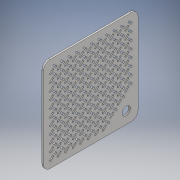
# Autodesk Inventor part: ExtrusionFrontpanel2
Saved by Autodesk Inventor 2017 (Build 210142000, 142)
## iProperties
Created: 2019-06-19
Part Number: ExtrusionFrontpanel2
Material: Generic
Document SubType Name: Modeling
Designer: DDeGo
Density: 1 g/cm^3
Appearance: Default
Author: DDeGo
Autodesk Inventor part; units mm, degrees
(part 1 of 3)
ref_plane "YZ Plane" through (0, 0, 0) normal (1, 0, 0) x (0, 1, 0)
ref_plane "XZ Plane" through (0, 0, 0) normal (0, 1, 0) x (-1, 0, 0)
ref_plane "XY Plane" through (0, 0, 0) normal (0, 0, 1) x (1, 0, 0)
sketch "Sketch1" plane through (0, 0, 0) normal (1, 0, 0) x (0, 1, 0)
  line L0 (0, 13) -> (157, 13)
  line L1 (170, 0) -> (170, -157)
  line L2 (157, -170) -> (0, -170)
  line L3 (-13, -157) -> (-13, 0)
  arc A0 (170, 0) -> (157, 13) centre (157, 0) ccw
  arc A1 (157, -170) -> (170, -157) centre (157, -157) ccw
  arc A2 (-13, -157) -> (0, -170) centre (0, -157) ccw
  arc A3 (0, 13) -> (-13, 0) centre (0, 0) ccw
  point P0 (-13, 13)
  dimension "d0" = 183
  dimension "d1" = 183
  dimension "d4" = 13
  constraints: 8 end point, 8 point on circle, 8 tangent, 4 centre point, 3 equal radius, 2 parallel, 2 point on line, 1 coincident, 1 horizontal, 1 perpendicular
  measures "d0" distance between parallel lines of L2 L0
  measures "d1" distance between parallel lines of L3 L1
  measures "d4" radius of A0
extrude "Extrusion1" add sketch "Sketch1" along normal blind 3
sketch "Sketch7" plane through (3, 0, 0) normal (1, 0, 0) x (0, 0, -1)
  arc A0 (170, 157) -> (157, 170) centre (157, 157) ccw construction
  line L0 (0, 0) -> (157, 0) construction
  line L1 (157, 0) -> (157, 157) construction
  line L2 (157, 157) -> (0, 157) construction
  line L3 (0, 157) -> (0, 0) construction
  line L4 (157, 0) -> (152, 5) construction
  line L5 (158.0607, 1.0607) -> (153.0607, 6.0607)
  line L6 (150.9393, 3.9393) -> (155.9393, -1.0607)
  arc A1 (155.9393, -1.0607) -> (158.0607, 1.0607) centre (157, 0) ccw
  arc A2 (153.0607, 6.0607) -> (150.9393, 3.9393) centre (152, 5) ccw
  line L7 (150.3787, 11.6213) -> (145.3787, 6.6213) construction
  line L8 (151.4393, 10.5607) -> (146.4393, 5.5607)
  line L9 (144.318, 7.682) -> (149.318, 12.682)
  arc A3 (151.4393, 10.5607) -> (149.318, 12.682) centre (150.3787, 11.6213) ccw
  arc A4 (144.318, 7.682) -> (146.4393, 5.5607) centre (145.3787, 6.6213) ccw
  line L10 (148.9393, 8.0607) -> (150.9393, 6.0607) construction
  line L11 (157, 14.5379) -> (152, 19.5379) construction
  line L12 (150.9393, 18.4772) -> (155.9393, 13.4772)
  arc A5 (155.9393, 13.4772) -> (158.0607, 15.5985) centre (157, 14.5379) ccw
  line L13 (158.0607, 15.5985) -> (153.0607, 20.5985)
  arc A6 (153.0607, 20.5985) -> (150.9393, 18.4772) centre (152, 19.5379) ccw
  line L14 (148.9393, 22.5985) -> (150.9393, 20.5985) construction
  line L15 (151.4393, 25.0985) -> (146.4393, 20.0985)
  arc A7 (144.318, 22.2198) -> (146.4393, 20.0985) centre (145.3787, 21.1592) ccw
  line L16 (150.3787, 26.1592) -> (145.3787, 21.1592) construction
  line L17 (144.318, 22.2198) -> (149.318, 27.2198)
  arc A8 (151.4393, 25.0985) -> (149.318, 27.2198) centre (150.3787, 26.1592) ccw
  line L18 (157, 29.0757) -> (152, 34.0757) construction
  line L19 (150.9393, 33.0151) -> (155.9393, 28.0151)
  arc A9 (155.9393, 28.0151) -> (158.0607, 30.1364) centre (157, 29.0757) ccw
  line L20 (158.0607, 30.1364) -> (153.0607, 35.1364)
  arc A10 (153.0607, 35.1364) -> (150.9393, 33.0151) centre (152, 34.0757) ccw
  line L21 (148.9393, 37.1364) -> (150.9393, 35.1364) construction
  line L22 (151.4393, 39.6364) -> (146.4393, 34.6364)
  arc A11 (144.318, 36.7577) -> (146.4393, 34.6364) centre (145.3787, 35.6971) ccw
  line L23 (150.3787, 40.6971) -> (145.3787, 35.6971) construction
  line L24 (144.318, 36.7577) -> (149.318, 41.7577)
  arc A12 (151.4393, 39.6364) -> (149.318, 41.7577) centre (150.3787, 40.6971) ccw
  line L25 (157, 43.6136) -> (152, 48.6136) construction
  line L26 (150.9393, 47.5529) -> (155.9393, 42.5529)
  arc A13 (155.9393, 42.5529) -> (158.0607, 44.6743) centre (157, 43.6136) ccw
  line L27 (158.0607, 44.6743) -> (153.0607, 49.6743)
  arc A14 (153.0607, 49.6743) -> (150.9393, 47.5529) centre (152, 48.6136) ccw
  line L28 (148.9393, 51.6743) -> (150.9393, 49.6743) construction
  line L29 (151.4393, 54.1743) -> (146.4393, 49.1743)
  arc A15 (144.318, 51.2956) -> (146.4393, 49.1743) centre (145.3787, 50.2349) ccw
  line L30 (150.3787, 55.2349) -> (145.3787, 50.2349) construction
  line L31 (144.318, 51.2956) -> (149.318, 56.2956)
  arc A16 (151.4393, 54.1743) -> (149.318, 56.2956) centre (150.3787, 55.2349) ccw
  line L32 (157, 58.1515) -> (152, 63.1515) construction
  line L33 (150.9393, 62.0908) -> (155.9393, 57.0908)
  arc A17 (155.9393, 57.0908) -> (158.0607, 59.2121) centre (157, 58.1515) ccw
  line L34 (158.0607, 59.2121) -> (153.0607, 64.2121)
  arc A18 (153.0607, 64.2121) -> (150.9393, 62.0908) centre (152, 63.1515) ccw
  line L35 (148.9393, 66.2121) -> (150.9393, 64.2121) construction
  line L36 (151.4393, 68.7121) -> (146.4393, 63.7121)
  arc A19 (144.318, 65.8335) -> (146.4393, 63.7121) centre (145.3787, 64.7728) ccw
  line L37 (150.3787, 69.7728) -> (145.3787, 64.7728) construction
  line L38 (144.318, 65.8335) -> (149.318, 70.8335)
  arc A20 (151.4393, 68.7121) -> (149.318, 70.8335) centre (150.3787, 69.7728) ccw
  line L39 (157, 72.6893) -> (152, 77.6893) construction
  line L40 (150.9393, 76.6287) -> (155.9393, 71.6287)
  arc A21 (155.9393, 71.6287) -> (158.0607, 73.75) centre (157, 72.6893) ccw
  line L41 (158.0607, 73.75) -> (153.0607, 78.75)
  arc A22 (153.0607, 78.75) -> (150.9393, 76.6287) centre (152, 77.6893) ccw
  line L42 (148.9393, 80.75) -> (150.9393, 78.75) construction
  line L43 (151.4393, 83.25) -> (146.4393, 78.25)
  arc A23 (144.318, 80.3713) -> (146.4393, 78.25) centre (145.3787, 79.3107) ccw
  line L44 (150.3787, 84.3107) -> (145.3787, 79.3107) construction
  line L45 (144.318, 80.3713) -> (149.318, 85.3713)
  arc A24 (151.4393, 83.25) -> (149.318, 85.3713) centre (150.3787, 84.3107) ccw
  line L46 (157, 87.2272) -> (152, 92.2272) construction
  line L47 (150.9393, 91.1665) -> (155.9393, 86.1665)
  arc A25 (155.9393, 86.1665) -> (158.0607, 88.2879) centre (157, 87.2272) ccw
  line L48 (158.0607, 88.2879) -> (153.0607, 93.2879)
  arc A26 (153.0607, 93.2879) -> (150.9393, 91.1665) centre (152, 92.2272) ccw
  line L49 (148.9393, 95.2879) -> (150.9393, 93.2879) construction
  line L50 (151.4393, 97.7879) -> (146.4393, 92.7879)
  arc A27 (144.318, 94.9092) -> (146.4393, 92.7879) centre (145.3787, 93.8485) ccw
  line L51 (150.3787, 98.8485) -> (145.3787, 93.8485) construction
  line L52 (144.318, 94.9092) -> (149.318, 99.9092)
  arc A28 (151.4393, 97.7879) -> (149.318, 99.9092) centre (150.3787, 98.8485) ccw
  line L53 (157, 101.7651) -> (152, 106.7651) construction
  line L54 (150.9393, 105.7044) -> (155.9393, 100.7044)
  arc A29 (155.9393, 100.7044) -> (158.0607, 102.8257) centre (157, 101.7651) ccw
  line L55 (158.0607, 102.8257) -> (153.0607, 107.8257)
  arc A30 (153.0607, 107.8257) -> (150.9393, 105.7044) centre (152, 106.7651) ccw
  line L56 (148.9393, 109.8257) -> (150.9393, 107.8257) construction
  line L57 (151.4393, 112.3257) -> (146.4393, 107.3257)
  arc A31 (144.318, 109.4471) -> (146.4393, 107.3257) centre (145.3787, 108.3864) ccw
  line L58 (150.3787, 113.3864) -> (145.3787, 108.3864) construction
  line L59 (144.318, 109.4471) -> (149.318, 114.4471)
  arc A32 (151.4393, 112.3257) -> (149.318, 114.4471) centre (150.3787, 113.3864) ccw
  line L60 (157, 116.3029) -> (152, 121.3029) construction
  line L61 (150.9393, 120.2423) -> (155.9393, 115.2423)
  arc A33 (155.9393, 115.2423) -> (158.0607, 117.3636) centre (157, 116.3029) ccw
  line L62 (158.0607, 117.3636) -> (153.0607, 122.3636)
  arc A34 (153.0607, 122.3636) -> (150.9393, 120.2423) centre (152, 121.3029) ccw
  line L63 (148.9393, 124.3636) -> (150.9393, 122.3636) construction
  line L64 (151.4393, 126.8636) -> (146.4393, 121.8636)
  arc A35 (144.318, 123.9849) -> (146.4393, 121.8636) centre (145.3787, 122.9243) ccw
  line L65 (150.3787, 127.9243) -> (145.3787, 122.9243) construction
  line L66 (144.318, 123.9849) -> (149.318, 128.9849)
  arc A36 (151.4393, 126.8636) -> (149.318, 128.9849) centre (150.3787, 127.9243) ccw
  line L67 (157, 130.8408) -> (152, 135.8408) construction
  line L68 (150.9393, 134.7802) -> (155.9393, 129.7802)
  arc A37 (155.9393, 129.7802) -> (158.0607, 131.9015) centre (157, 130.8408) ccw
  line L69 (158.0607, 131.9015) -> (153.0607, 136.9015)
  arc A38 (153.0607, 136.9015) -> (150.9393, 134.7802) centre (152, 135.8408) ccw
  line L70 (148.9393, 138.9015) -> (150.9393, 136.9015) construction
  line L71 (151.4393, 141.4015) -> (146.4393, 136.4015)
  arc A39 (144.318, 138.5228) -> (146.4393, 136.4015) centre (145.3787, 137.4621) ccw
  line L72 (150.3787, 142.4621) -> (145.3787, 137.4621) construction
  line L73 (144.318, 138.5228) -> (149.318, 143.5228)
  arc A40 (151.4393, 141.4015) -> (149.318, 143.5228) centre (150.3787, 142.4621) ccw
  line L74 (157, 145.3787) -> (152, 150.3787) construction
  line L75 (150.9393, 149.318) -> (155.9393, 144.318)
  arc A41 (155.9393, 144.318) -> (158.0607, 146.4393) centre (157, 145.3787) ccw
  line L76 (158.0607, 146.4393) -> (153.0607, 151.4393)
  arc A42 (153.0607, 151.4393) -> (150.9393, 149.318) centre (152, 150.3787) ccw
  line L77 (148.9393, 153.4393) -> (150.9393, 151.4393) construction
  line L78 (151.4393, 155.9393) -> (146.4393, 150.9393)
  arc A43 (144.318, 153.0607) -> (146.4393, 150.9393) centre (145.3787, 152) ccw
  line L79 (150.3787, 157) -> (145.3787, 152) construction
  line L80 (144.318, 153.0607) -> (149.318, 158.0607)
  arc A44 (151.4393, 155.9393) -> (149.318, 158.0607) centre (150.3787, 157) ccw
  line L81 (142.4621, 0) -> (137.4621, 5) construction
  line L82 (136.4015, 3.9393) -> (141.4015, -1.0607)
  arc A45 (141.4015, -1.0607) -> (143.5228, 1.0607) centre (142.4621, 0) ccw
  line L83 (143.5228, 1.0607) -> (138.5228, 6.0607)
  arc A46 (138.5228, 6.0607) -> (136.4015, 3.9393) centre (137.4621, 5) ccw
  line L84 (134.4015, 8.0607) -> (136.4015, 6.0607) construction
  line L85 (136.9015, 10.5607) -> (131.9015, 5.5607)
  arc A47 (129.7802, 7.682) -> (131.9015, 5.5607) centre (130.8408, 6.6213) ccw
  line L86 (135.8408, 11.6213) -> (130.8408, 6.6213) construction
  line L87 (129.7802, 7.682) -> (134.7802, 12.682)
  arc A48 (136.9015, 10.5607) -> (134.7802, 12.682) centre (135.8408, 11.6213) ccw
  line L88 (142.4621, 14.5379) -> (137.4621, 19.5379) construction
  line L89 (136.4015, 18.4772) -> (141.4015, 13.4772)
  arc A49 (141.4015, 13.4772) -> (143.5228, 15.5985) centre (142.4621, 14.5379) ccw
  line L90 (143.5228, 15.5985) -> (138.5228, 20.5985)
  arc A50 (138.5228, 20.5985) -> (136.4015, 18.4772) centre (137.4621, 19.5379) ccw
  line L91 (134.4015, 22.5985) -> (136.4015, 20.5985) construction
  line L92 (136.9015, 25.0985) -> (131.9015, 20.0985)
  arc A51 (129.7802, 22.2198) -> (131.9015, 20.0985) centre (130.8408, 21.1592) ccw
  line L93 (135.8408, 26.1592) -> (130.8408, 21.1592) construction
  line L94 (129.7802, 22.2198) -> (134.7802, 27.2198)
  arc A52 (136.9015, 25.0985) -> (134.7802, 27.2198) centre (135.8408, 26.1592) ccw
  line L95 (142.4621, 29.0757) -> (137.4621, 34.0757) construction
  line L96 (136.4015, 33.0151) -> (141.4015, 28.0151)
  arc A53 (141.4015, 28.0151) -> (143.5228, 30.1364) centre (142.4621, 29.0757) ccw
  line L97 (143.5228, 30.1364) -> (138.5228, 35.1364)
  arc A54 (138.5228, 35.1364) -> (136.4015, 33.0151) centre (137.4621, 34.0757) ccw
  line L98 (134.4015, 37.1364) -> (136.4015, 35.1364) construction
  line L99 (136.9015, 39.6364) -> (131.9015, 34.6364)
  arc A55 (129.7802, 36.7577) -> (131.9015, 34.6364) centre (130.8408, 35.6971) ccw
  line L100 (135.8408, 40.6971) -> (130.8408, 35.6971) construction
  line L101 (129.7802, 36.7577) -> (134.7802, 41.7577)
  arc A56 (136.9015, 39.6364) -> (134.7802, 41.7577) centre (135.8408, 40.6971) ccw
  line L102 (142.4621, 43.6136) -> (137.4621, 48.6136) construction
  line L103 (136.4015, 47.5529) -> (141.4015, 42.5529)
  arc A57 (141.4015, 42.5529) -> (143.5228, 44.6743) centre (142.4621, 43.6136) ccw
  line L104 (143.5228, 44.6743) -> (138.5228, 49.6743)
  arc A58 (138.5228, 49.6743) -> (136.4015, 47.5529) centre (137.4621, 48.6136) ccw
  line L105 (134.4015, 51.6743) -> (136.4015, 49.6743) construction
  line L106 (136.9015, 54.1743) -> (131.9015, 49.1743)
  arc A59 (129.7802, 51.2956) -> (131.9015, 49.1743) centre (130.8408, 50.2349) ccw
  line L107 (135.8408, 55.2349) -> (130.8408, 50.2349) construction
  line L108 (129.7802, 51.2956) -> (134.7802, 56.2956)
  arc A60 (136.9015, 54.1743) -> (134.7802, 56.2956) centre (135.8408, 55.2349) ccw
  line L109 (142.4621, 58.1515) -> (137.4621, 63.1515) construction
  line L110 (136.4015, 62.0908) -> (141.4015, 57.0908)
  arc A61 (141.4015, 57.0908) -> (143.5228, 59.2121) centre (142.4621, 58.1515) ccw
  line L111 (143.5228, 59.2121) -> (138.5228, 64.2121)
  arc A62 (138.5228, 64.2121) -> (136.4015, 62.0908) centre (137.4621, 63.1515) ccw
  line L112 (134.4015, 66.2121) -> (136.4015, 64.2121) construction
  line L113 (136.9015, 68.7121) -> (131.9015, 63.7121)
  arc A63 (129.7802, 65.8335) -> (131.9015, 63.7121) centre (130.8408, 64.7728) ccw
  line L114 (135.8408, 69.7728) -> (130.8408, 64.7728) construction
  line L115 (129.7802, 65.8335) -> (134.7802, 70.8335)
  arc A64 (136.9015, 68.7121) -> (134.7802, 70.8335) centre (135.8408, 69.7728) ccw
  line L116 (142.4621, 72.6893) -> (137.4621, 77.6893) construction
  line L117 (136.4015, 76.6287) -> (141.4015, 71.6287)
  arc A65 (141.4015, 71.6287) -> (143.5228, 73.75) centre (142.4621, 72.6893) ccw
  line L118 (143.5228, 73.75) -> (138.5228, 78.75)
  arc A66 (138.5228, 78.75) -> (136.4015, 76.6287) centre (137.4621, 77.6893) ccw
  line L119 (134.4015, 80.75) -> (136.4015, 78.75) construction
  line L120 (136.9015, 83.25) -> (131.9015, 78.25)
  arc A67 (129.7802, 80.3713) -> (131.9015, 78.25) centre (130.8408, 79.3107) ccw
  line L121 (135.8408, 84.3107) -> (130.8408, 79.3107) construction
  line L122 (129.7802, 80.3713) -> (134.7802, 85.3713)
  arc A68 (136.9015, 83.25) -> (134.7802, 85.3713) centre (135.8408, 84.3107) ccw
  line L123 (142.4621, 87.2272) -> (137.4621, 92.2272) construction
  line L124 (136.4015, 91.1665) -> (141.4015, 86.1665)
  arc A69 (141.4015, 86.1665) -> (143.5228, 88.2879) centre (142.4621, 87.2272) ccw
  line L125 (143.5228, 88.2879) -> (138.5228, 93.2879)
  arc A70 (138.5228, 93.2879) -> (136.4015, 91.1665) centre (137.4621, 92.2272) ccw
  line L126 (134.4015, 95.2879) -> (136.4015, 93.2879) construction
  line L127 (136.9015, 97.7879) -> (131.9015, 92.7879)
  arc A71 (129.7802, 94.9092) -> (131.9015, 92.7879) centre (130.8408, 93.8485) ccw
  line L128 (135.8408, 98.8485) -> (130.8408, 93.8485) construction
  line L129 (129.7802, 94.9092) -> (134.7802, 99.9092)
  arc A72 (136.9015, 97.7879) -> (134.7802, 99.9092) centre (135.8408, 98.8485) ccw
  line L130 (142.4621, 101.7651) -> (137.4621, 106.7651) construction
  line L131 (136.4015, 105.7044) -> (141.4015, 100.7044)
  arc A73 (141.4015, 100.7044) -> (143.5228, 102.8257) centre (142.4621, 101.7651) ccw
  line L132 (143.5228, 102.8257) -> (138.5228, 107.8257)
  arc A74 (138.5228, 107.8257) -> (136.4015, 105.7044) centre (137.4621, 106.7651) ccw
  line L133 (134.4015, 109.8257) -> (136.4015, 107.8257) construction
  line L134 (136.9015, 112.3257) -> (131.9015, 107.3257)
  arc A75 (129.7802, 109.4471) -> (131.9015, 107.3257) centre (130.8408, 108.3864) ccw
  line L135 (135.8408, 113.3864) -> (130.8408, 108.3864) construction
  line L136 (129.7802, 109.4471) -> (134.7802, 114.4471)
  arc A76 (136.9015, 112.3257) -> (134.7802, 114.4471) centre (135.8408, 113.3864) ccw
  line L137 (142.4621, 116.3029) -> (137.4621, 121.3029) construction
  line L138 (136.4015, 120.2423) -> (141.4015, 115.2423)
  arc A77 (141.4015, 115.2423) -> (143.5228, 117.3636) centre (142.4621, 116.3029) ccw
  line L139 (143.5228, 117.3636) -> (138.5228, 122.3636)
  arc A78 (138.5228, 122.3636) -> (136.4015, 120.2423) centre (137.4621, 121.3029) ccw
  line L140 (134.4015, 124.3636) -> (136.4015, 122.3636) construction
  line L141 (136.9015, 126.8636) -> (131.9015, 121.8636)
  arc A79 (129.7802, 123.9849) -> (131.9015, 121.8636) centre (130.8408, 122.9243) ccw
  line L142 (135.8408, 127.9243) -> (130.8408, 122.9243) construction
  line L143 (129.7802, 123.9849) -> (134.7802, 128.9849)
  arc A80 (136.9015, 126.8636) -> (134.7802, 128.9849) centre (135.8408, 127.9243) ccw
  line L144 (142.4621, 130.8408) -> (137.4621, 135.8408) construction
  line L145 (136.4015, 134.7802) -> (141.4015, 129.7802)
  arc A81 (141.4015, 129.7802) -> (143.5228, 131.9015) centre (142.4621, 130.8408) ccw
  line L146 (143.5228, 131.9015) -> (138.5228, 136.9015)
  arc A82 (138.5228, 136.9015) -> (136.4015, 134.7802) centre (137.4621, 135.8408) ccw
  line L147 (134.4015, 138.9015) -> (136.4015, 136.9015) construction
  line L148 (136.9015, 141.4015) -> (131.9015, 136.4015)
  arc A83 (129.7802, 138.5228) -> (131.9015, 136.4015) centre (130.8408, 137.4621) ccw
  line L149 (135.8408, 142.4621) -> (130.8408, 137.4621) construction
  line L150 (129.7802, 138.5228) -> (134.7802, 143.5228)
  arc A84 (136.9015, 141.4015) -> (134.7802, 143.5228) centre (135.8408, 142.4621) ccw
  line L151 (142.4621, 145.3787) -> (137.4621, 150.3787) construction
  line L152 (136.4015, 149.318) -> (141.4015, 144.318)
  arc A85 (141.4015, 144.318) -> (143.5228, 146.4393) centre (142.4621, 145.3787) ccw
  line L153 (143.5228, 146.4393) -> (138.5228, 151.4393)
  arc A86 (138.5228, 151.4393) -> (136.4015, 149.318) centre (137.4621, 150.3787) ccw
  line L154 (134.4015, 153.4393) -> (136.4015, 151.4393) construction
  line L155 (136.9015, 155.9393) -> (131.9015, 150.9393)
  arc A87 (129.7802, 153.0607) -> (131.9015, 150.9393) centre (130.8408, 152) ccw
  line L156 (135.8408, 157) -> (130.8408, 152) construction
  line L157 (129.7802, 153.0607) -> (134.7802, 158.0607)
  arc A88 (136.9015, 155.9393) -> (134.7802, 158.0607) centre (135.8408, 157) ccw
  line L158 (127.9243, 0) -> (122.9243, 5) construction
  line L159 (121.8636, 3.9393) -> (126.8636, -1.0607)
  arc A89 (126.8636, -1.0607) -> (128.9849, 1.0607) centre (127.9243, 0) ccw
  line L160 (128.9849, 1.0607) -> (123.9849, 6.0607)
  arc A90 (123.9849, 6.0607) -> (121.8636, 3.9393) centre (122.9243, 5) ccw
  line L161 (119.8636, 8.0607) -> (121.8636, 6.0607) construction
  line L162 (122.3636, 10.5607) -> (117.3636, 5.5607)
  arc A91 (115.2423, 7.682) -> (117.3636, 5.5607) centre (116.3029, 6.6213) ccw
  line L163 (121.3029, 11.6213) -> (116.3029, 6.6213) construction
  line L164 (115.2423, 7.682) -> (120.2423, 12.682)
  arc A92 (122.3636, 10.5607) -> (120.2423, 12.682) centre (121.3029, 11.6213) ccw
  line L165 (127.9243, 14.5379) -> (122.9243, 19.5379) construction
  line L166 (121.8636, 18.4772) -> (126.8636, 13.4772)
  arc A93 (126.8636, 13.4772) -> (128.9849, 15.5985) centre (127.9243, 14.5379) ccw
  line L167 (128.9849, 15.5985) -> (123.9849, 20.5985)
  arc A94 (123.9849, 20.5985) -> (121.8636, 18.4772) centre (122.9243, 19.5379) ccw
  line L168 (119.8636, 22.5985) -> (121.8636, 20.5985) construction
  line L169 (122.3636, 25.0985) -> (117.3636, 20.0985)
  arc A95 (115.2423, 22.2198) -> (117.3636, 20.0985) centre (116.3029, 21.1592) ccw
  line L170 (121.3029, 26.1592) -> (116.3029, 21.1592) construction
  line L171 (115.2423, 22.2198) -> (120.2423, 27.2198)
  arc A96 (122.3636, 25.0985) -> (120.2423, 27.2198) centre (121.3029, 26.1592) ccw
  line L172 (127.9243, 29.0757) -> (122.9243, 34.0757) construction
  line L173 (121.8636, 33.0151) -> (126.8636, 28.0151)
  arc A97 (126.8636, 28.0151) -> (128.9849, 30.1364) centre (127.9243, 29.0757) ccw
  line L174 (128.9849, 30.1364) -> (123.9849, 35.1364)
  arc A98 (123.9849, 35.1364) -> (121.8636, 33.0151) centre (122.9243, 34.0757) ccw
  line L175 (119.8636, 37.1364) -> (121.8636, 35.1364) construction
  line L176 (122.3636, 39.6364) -> (117.3636, 34.6364)
  arc A99 (115.2423, 36.7577) -> (117.3636, 34.6364) centre (116.3029, 35.6971) ccw
  line L177 (121.3029, 40.6971) -> (116.3029, 35.6971) construction
  line L178 (115.2423, 36.7577) -> (120.2423, 41.7577)
  arc A100 (122.3636, 39.6364) -> (120.2423, 41.7577) centre (121.3029, 40.6971) ccw
  line L179 (127.9243, 43.6136) -> (122.9243, 48.6136) construction
  line L180 (121.8636, 47.5529) -> (126.8636, 42.5529)
  arc A101 (126.8636, 42.5529) -> (128.9849, 44.6743) centre (127.9243, 43.6136) ccw
  line L181 (128.9849, 44.6743) -> (123.9849, 49.6743)
  arc A102 (123.9849, 49.6743) -> (121.8636, 47.5529) centre (122.9243, 48.6136) ccw
  line L182 (119.8636, 51.6743) -> (121.8636, 49.6743) construction
  line L183 (122.3636, 54.1743) -> (117.3636, 49.1743)
  arc A103 (115.2423, 51.2956) -> (117.3636, 49.1743) centre (116.3029, 50.2349) ccw
  line L184 (121.3029, 55.2349) -> (116.3029, 50.2349) construction
  line L185 (115.2423, 51.2956) -> (120.2423, 56.2956)
  arc A104 (122.3636, 54.1743) -> (120.2423, 56.2956) centre (121.3029, 55.2349) ccw
  line L186 (127.9243, 58.1515) -> (122.9243, 63.1515) construction
  line L187 (121.8636, 62.0908) -> (126.8636, 57.0908)
  arc A105 (126.8636, 57.0908) -> (128.9849, 59.2121) centre (127.9243, 58.1515) ccw
  line L188 (128.9849, 59.2121) -> (123.9849, 64.2121)
  arc A106 (123.9849, 64.2121) -> (121.8636, 62.0908) centre (122.9243, 63.1515) ccw
  line L189 (119.8636, 66.2121) -> (121.8636, 64.2121) construction
  line L190 (122.3636, 68.7121) -> (117.3636, 63.7121)
  arc A107 (115.2423, 65.8335) -> (117.3636, 63.7121) centre (116.3029, 64.7728) ccw
  line L191 (121.3029, 69.7728) -> (116.3029, 64.7728) construction
  line L192 (115.2423, 65.8335) -> (120.2423, 70.8335)
  arc A108 (122.3636, 68.7121) -> (120.2423, 70.8335) centre (121.3029, 69.7728) ccw
  line L193 (127.9243, 72.6893) -> (122.9243, 77.6893) construction
  line L194 (121.8636, 76.6287) -> (126.8636, 71.6287)
  arc A109 (126.8636, 71.6287) -> (128.9849, 73.75) centre (127.9243, 72.6893) ccw
  line L195 (128.9849, 73.75) -> (123.9849, 78.75)
  arc A110 (123.9849, 78.75) -> (121.8636, 76.6287) centre (122.9243, 77.6893) ccw
  line L196 (119.8636, 80.75) -> (121.8636, 78.75) construction
  line L197 (122.3636, 83.25) -> (117.3636, 78.25)
  arc A111 (115.2423, 80.3713) -> (117.3636, 78.25) centre (116.3029, 79.3107) ccw
  line L198 (121.3029, 84.3107) -> (116.3029, 79.3107) construction
  line L199 (115.2423, 80.3713) -> (120.2423, 85.3713)
  arc A112 (122.3636, 83.25) -> (120.2423, 85.3713) centre (121.3029, 84.3107) ccw
  line L200 (127.9243, 87.2272) -> (122.9243, 92.2272) construction
  line L201 (121.8636, 91.1665) -> (126.8636, 86.1665)
  arc A113 (126.8636, 86.1665) -> (128.9849, 88.2879) centre (127.9243, 87.2272) ccw
  line L202 (128.9849, 88.2879) -> (123.9849, 93.2879)
  arc A114 (123.9849, 93.2879) -> (121.8636, 91.1665) centre (122.9243, 92.2272) ccw
  line L203 (119.8636, 95.2879) -> (121.8636, 93.2879) construction
  line L204 (122.3636, 97.7879) -> (117.3636, 92.7879)
  arc A115 (115.2423, 94.9092) -> (117.3636, 92.7879) centre (116.3029, 93.8485) ccw
  line L205 (121.3029, 98.8485) -> (116.3029, 93.8485) construction
  line L206 (115.2423, 94.9092) -> (120.2423, 99.9092)
  arc A116 (122.3636, 97.7879) -> (120.2423, 99.9092) centre (121.3029, 98.8485) ccw
  line L207 (127.9243, 101.7651) -> (122.9243, 106.7651) construction
  line L208 (121.8636, 105.7044) -> (126.8636, 100.7044)
  arc A117 (126.8636, 100.7044) -> (128.9849, 102.8257) centre (127.9243, 101.7651) ccw
  line L209 (128.9849, 102.8257) -> (123.9849, 107.8257)
  arc A118 (123.9849, 107.8257) -> (121.8636, 105.7044) centre (122.9243, 106.7651) ccw
  line L210 (119.8636, 109.8257) -> (121.8636, 107.8257) construction
  line L211 (122.3636, 112.3257) -> (117.3636, 107.3257)
  arc A119 (115.2423, 109.4471) -> (117.3636, 107.3257) centre (116.3029, 108.3864) ccw
  line L212 (121.3029, 113.3864) -> (116.3029, 108.3864) construction
  line L213 (115.2423, 109.4471) -> (120.2423, 114.4471)
  arc A120 (122.3636, 112.3257) -> (120.2423, 114.4471) centre (121.3029, 113.3864) ccw
  line L214 (127.9243, 116.3029) -> (122.9243, 121.3029) construction
  line L215 (121.8636, 120.2423) -> (126.8636, 115.2423)
  arc A121 (126.8636, 115.2423) -> (128.9849, 117.3636) centre (127.9243, 116.3029) ccw
  line L216 (128.9849, 117.3636) -> (123.9849, 122.3636)
  arc A122 (123.9849, 122.3636) -> (121.8636, 120.2423) centre (122.9243, 121.3029) ccw
  line L217 (119.8636, 124.3636) -> (121.8636, 122.3636) construction
  line L218 (122.3636, 126.8636) -> (117.3636, 121.8636)
  arc A123 (115.2423, 123.9849) -> (117.3636, 121.8636) centre (116.3029, 122.9243) ccw
  line L219 (121.3029, 127.9243) -> (116.3029, 122.9243) construction
  line L220 (115.2423, 123.9849) -> (120.2423, 128.9849)
  arc A124 (122.3636, 126.8636) -> (120.2423, 128.9849) centre (121.3029, 127.9243) ccw
  line L221 (127.9243, 130.8408) -> (122.9243, 135.8408) construction
  line L222 (121.8636, 134.7802) -> (126.8636, 129.7802)
  arc A125 (126.8636, 129.7802) -> (128.9849, 131.9015) centre (127.9243, 130.8408) ccw
  line L223 (128.9849, 131.9015) -> (123.9849, 136.9015)
  arc A126 (123.9849, 136.9015) -> (121.8636, 134.7802) centre (122.9243, 135.8408) ccw
  line L224 (119.8636, 138.9015) -> (121.8636, 136.9015) construction
  line L225 (122.3636, 141.4015) -> (117.3636, 136.4015)
  arc A127 (115.2423, 138.5228) -> (117.3636, 136.4015) centre (116.3029, 137.4621) ccw
  line L226 (121.3029, 142.4621) -> (116.3029, 137.4621) construction
  line L227 (115.2423, 138.5228) -> (120.2423, 143.5228)
  arc A128 (122.3636, 141.4015) -> (120.2423, 143.5228) centre (121.3029, 142.4621) ccw
  line L228 (127.9243, 145.3787) -> (122.9243, 150.3787) construction
  line L229 (121.8636, 149.318) -> (126.8636, 144.318)
  arc A129 (126.8636, 144.318) -> (128.9849, 146.4393) centre (127.9243, 145.3787) ccw
  line L230 (128.9849, 146.4393) -> (123.9849, 151.4393)
  arc A130 (123.9849, 151.4393) -> (121.8636, 149.318) centre (122.9243, 150.3787) ccw
  line L231 (119.8636, 153.4393) -> (121.8636, 151.4393) construction
  line L232 (122.3636, 155.9393) -> (117.3636, 150.9393)
  arc A131 (115.2423, 153.0607) -> (117.3636, 150.9393) centre (116.3029, 152) ccw
  line L233 (121.3029, 157) -> (116.3029, 152) construction
  line L234 (115.2423, 153.0607) -> (120.2423, 158.0607)
  arc A132 (122.3636, 155.9393) -> (120.2423, 158.0607) centre (121.3029, 157) ccw
  line L235 (113.3864, 0) -> (108.3864, 5) construction
  line L236 (107.3257, 3.9393) -> (112.3257, -1.0607)
  arc A133 (112.3257, -1.0607) -> (114.4471, 1.0607) centre (113.3864, 0) ccw
  line L237 (114.4471, 1.0607) -> (109.4471, 6.0607)
  arc A134 (109.4471, 6.0607) -> (107.3257, 3.9393) centre (108.3864, 5) ccw
  line L238 (105.3257, 8.0607) -> (107.3257, 6.0607) construction
  line L239 (107.8257, 10.5607) -> (102.8257, 5.5607)
  arc A135 (100.7044, 7.682) -> (102.8257, 5.5607) centre (101.7651, 6.6213) ccw
  line L240 (106.7651, 11.6213) -> (101.7651, 6.6213) construction
  line L241 (100.7044, 7.682) -> (105.7044, 12.682)
  arc A136 (107.8257, 10.5607) -> (105.7044, 12.682) centre (106.7651, 11.6213) ccw
  line L242 (113.3864, 14.5379) -> (108.3864, 19.5379) construction
  line L243 (107.3257, 18.4772) -> (112.3257, 13.4772)
  arc A137 (112.3257, 13.4772) -> (114.4471, 15.5985) centre (113.3864, 14.5379) ccw
  line L244 (114.4471, 15.5985) -> (109.4471, 20.5985)
  arc A138 (109.4471, 20.5985) -> (107.3257, 18.4772) centre (108.3864, 19.5379) ccw
  line L245 (105.3257, 22.5985) -> (107.3257, 20.5985) construction
  line L246 (107.8257, 25.0985) -> (102.8257, 20.0985)
  arc A139 (100.7044, 22.2198) -> (102.8257, 20.0985) centre (101.7651, 21.1592) ccw
  line L247 (106.7651, 26.1592) -> (101.7651, 21.1592) construction
  line L248 (100.7044, 22.2198) -> (105.7044, 27.2198)
  arc A140 (107.8257, 25.0985) -> (105.7044, 27.2198) centre (106.7651, 26.1592) ccw
  line L249 (113.3864, 29.0757) -> (108.3864, 34.0757) construction
  line L250 (107.3257, 33.0151) -> (112.3257, 28.0151)
  arc A141 (112.3257, 28.0151) -> (114.4471, 30.1364) centre (113.3864, 29.0757) ccw
  line L251 (114.4471, 30.1364) -> (109.4471, 35.1364)
  arc A142 (109.4471, 35.1364) -> (107.3257, 33.0151) centre (108.3864, 34.0757) ccw
  line L252 (105.3257, 37.1364) -> (107.3257, 35.1364) construction
  line L253 (107.8257, 39.6364) -> (102.8257, 34.6364)
  arc A143 (100.7044, 36.7577) -> (102.8257, 34.6364) centre (101.7651, 35.6971) ccw
  line L254 (106.7651, 40.6971) -> (101.7651, 35.6971) construction
  line L255 (100.7044, 36.7577) -> (105.7044, 41.7577)
  arc A144 (107.8257, 39.6364) -> (105.7044, 41.7577) centre (106.7651, 40.6971) ccw
  line L256 (113.3864, 43.6136) -> (108.3864, 48.6136) construction
  line L257 (107.3257, 47.5529) -> (112.3257, 42.5529)
  arc A145 (112.3257, 42.5529) -> (114.4471, 44.6743) centre (113.3864, 43.6136) ccw
  line L258 (114.4471, 44.6743) -> (109.4471, 49.6743)
  arc A146 (109.4471, 49.6743) -> (107.3257, 47.5529) centre (108.3864, 48.6136) ccw
  line L259 (105.3257, 51.6743) -> (107.3257, 49.6743) construction
  line L260 (107.8257, 54.1743) -> (102.8257, 49.1743)
  arc A147 (100.7044, 51.2956) -> (102.8257, 49.1743) centre (101.7651, 50.2349) ccw
  line L261 (106.7651, 55.2349) -> (101.7651, 50.2349) construction
  line L262 (100.7044, 51.2956) -> (105.7044, 56.2956)
  arc A148 (107.8257, 54.1743) -> (105.7044, 56.2956) centre (106.7651, 55.2349) ccw
  line L263 (113.3864, 58.1515) -> (108.3864, 63.1515) construction
  line L264 (107.3257, 62.0908) -> (112.3257, 57.0908)
  arc A149 (112.3257, 57.0908) -> (114.4471, 59.2121) centre (113.3864, 58.1515) ccw
  line L265 (114.4471, 59.2121) -> (109.4471, 64.2121)
  arc A150 (109.4471, 64.2121) -> (107.3257, 62.0908) centre (108.3864, 63.1515) ccw
  line L266 (105.3257, 66.2121) -> (107.3257, 64.2121) construction
  line L267 (107.8257, 68.7121) -> (102.8257, 63.7121)
  arc A151 (100.7044, 65.8335) -> (102.8257, 63.7121) centre (101.7651, 64.7728) ccw
  line L268 (106.7651, 69.7728) -> (101.7651, 64.7728) construction
  line L269 (100.7044, 65.8335) -> (105.7044, 70.8335)
  arc A152 (107.8257, 68.7121) -> (105.7044, 70.8335) centre (106.7651, 69.7728) ccw
  line L270 (113.3864, 72.6893) -> (108.3864, 77.6893) construction
  line L271 (107.3257, 76.6287) -> (112.3257, 71.6287)
  arc A153 (112.3257, 71.6287) -> (114.4471, 73.75) centre (113.3864, 72.6893) ccw
  line L272 (114.4471, 73.75) -> (109.4471, 78.75)
  arc A154 (109.4471, 78.75) -> (107.3257, 76.6287) centre (108.3864, 77.6893) ccw
  line L273 (105.3257, 80.75) -> (107.3257, 78.75) construction
  line L274 (107.8257, 83.25) -> (102.8257, 78.25)
  arc A155 (100.7044, 80.3713) -> (102.8257, 78.25) centre (101.7651, 79.3107) ccw
  line L275 (106.7651, 84.3107) -> (101.7651, 79.3107) construction
  line L276 (100.7044, 80.3713) -> (105.7044, 85.3713)
  arc A156 (107.8257, 83.25) -> (105.7044, 85.3713) centre (106.7651, 84.3107) ccw
  line L277 (113.3864, 87.2272) -> (108.3864, 92.2272) construction
  line L278 (107.3257, 91.1665) -> (112.3257, 86.1665)
  arc A157 (112.3257, 86.1665) -> (114.4471, 88.2879) centre (113.3864, 87.2272) ccw
  line L279 (114.4471, 88.2879) -> (109.4471, 93.2879)
  arc A158 (109.4471, 93.2879) -> (107.3257, 91.1665) centre (108.3864, 92.2272) ccw
  line L280 (105.3257, 95.2879) -> (107.3257, 93.2879) construction
  line L281 (107.8257, 97.7879) -> (102.8257, 92.7879)
  arc A159 (100.7044, 94.9092) -> (102.8257, 92.7879) centre (101.7651, 93.8485) ccw
  line L282 (106.7651, 98.8485) -> (101.7651, 93.8485) construction
  line L283 (100.7044, 94.9092) -> (105.7044, 99.9092)
  arc A160 (107.8257, 97.7879) -> (105.7044, 99.9092) centre (106.7651, 98.8485) ccw
  line L284 (113.3864, 101.7651) -> (108.3864, 106.7651) construction
  line L285 (107.3257, 105.7044) -> (112.3257, 100.7044)
  arc A161 (112.3257, 100.7044) -> (114.4471, 102.8257) centre (113.3864, 101.7651) ccw
  line L286 (114.4471, 102.8257) -> (109.4471, 107.8257)
  arc A162 (109.4471, 107.8257) -> (107.3257, 105.7044) centre (108.3864, 106.7651) ccw
  line L287 (105.3257, 109.8257) -> (107.3257, 107.8257) construction
  line L288 (107.8257, 112.3257) -> (102.8257, 107.3257)
  arc A163 (100.7044, 109.4471) -> (102.8257, 107.3257) centre (101.7651, 108.3864) ccw
  line L289 (106.7651, 113.3864) -> (101.7651, 108.3864) construction
  line L290 (100.7044, 109.4471) -> (105.7044, 114.4471)
  arc A164 (107.8257, 112.3257) -> (105.7044, 114.4471) centre (106.7651, 113.3864) ccw
  line L291 (113.3864, 116.3029) -> (108.3864, 121.3029) construction
  line L292 (107.3257, 120.2423) -> (112.3257, 115.2423)
  arc A165 (112.3257, 115.2423) -> (114.4471, 117.3636) centre (113.3864, 116.3029) ccw
  line L293 (114.4471, 117.3636) -> (109.4471, 122.3636)
  arc A166 (109.4471, 122.3636) -> (107.3257, 120.2423) centre (108.3864, 121.3029) ccw
  line L294 (105.3257, 124.3636) -> (107.3257, 122.3636) construction
  line L295 (107.8257, 126.8636) -> (102.8257, 121.8636)
  arc A167 (100.7044, 123.9849) -> (102.8257, 121.8636) centre (101.7651, 122.9243) ccw
  line L296 (106.7651, 127.9243) -> (101.7651, 122.9243) construction
  line L297 (100.7044, 123.9849) -> (105.7044, 128.9849)
  arc A168 (107.8257, 126.8636) -> (105.7044, 128.9849) centre (106.7651, 127.9243) ccw
  line L298 (113.3864, 130.8408) -> (108.3864, 135.8408) construction
  line L299 (107.3257, 134.7802) -> (112.3257, 129.7802)
  arc A169 (112.3257, 129.7802) -> (114.4471, 131.9015) centre (113.3864, 130.8408) ccw
  line L300 (114.4471, 131.9015) -> (109.4471, 136.9015)
  arc A170 (109.4471, 136.9015) -> (107.3257, 134.7802) centre (108.3864, 135.8408) ccw
  line L301 (105.3257, 138.9015) -> (107.3257, 136.9015) construction
  line L302 (107.8257, 141.4015) -> (102.8257, 136.4015)
  arc A171 (100.7044, 138.5228) -> (102.8257, 136.4015) centre (101.7651, 137.4621) ccw
  line L303 (106.7651, 142.4621) -> (101.7651, 137.4621) construction
  line L304 (100.7044, 138.5228) -> (105.7044, 143.5228)
  arc A172 (107.8257, 141.4015) -> (105.7044, 143.5228) centre (106.7651, 142.4621) ccw
  line L305 (113.3864, 145.3787) -> (108.3864, 150.3787) construction
  line L306 (107.3257, 149.318) -> (112.3257, 144.318)
  arc A173 (112.3257, 144.318) -> (114.4471, 146.4393) centre (113.3864, 145.3787) ccw
  line L307 (114.4471, 146.4393) -> (109.4471, 151.4393)
  arc A174 (109.4471, 151.4393) -> (107.3257, 149.318) centre (108.3864, 150.3787) ccw
  line L308 (105.3257, 153.4393) -> (107.3257, 151.4393) construction
  line L309 (107.8257, 155.9393) -> (102.8257, 150.9393)
  arc A175 (100.7044, 153.0607) -> (102.8257, 150.9393) centre (101.7651, 152) ccw
  line L310 (106.7651, 157) -> (101.7651, 152) construction
  line L311 (100.7044, 153.0607) -> (105.7044, 158.0607)
  arc A176 (107.8257, 155.9393) -> (105.7044, 158.0607) centre (106.7651, 157) ccw
  line L312 (98.8485, 0) -> (93.8485, 5) construction
  line L313 (92.7879, 3.9393) -> (97.7879, -1.0607)
  arc A177 (97.7879, -1.0607) -> (99.9092, 1.0607) centre (98.8485, 0) ccw
  line L314 (99.9092, 1.0607) -> (94.9092, 6.0607)
  arc A178 (94.9092, 6.0607) -> (92.7879, 3.9393) centre (93.8485, 5) ccw
  line L315 (90.7879, 8.0607) -> (92.7879, 6.0607) construction
  line L316 (93.2879, 10.5607) -> (88.2879, 5.5607)
  arc A179 (86.1665, 7.682) -> (88.2879, 5.5607) centre (87.2272, 6.6213) ccw
  line L317 (92.2272, 11.6213) -> (87.2272, 6.6213) construction
  line L318 (86.1665, 7.682) -> (91.1665, 12.682)
  arc A180 (93.2879, 10.5607) -> (91.1665, 12.682) centre (92.2272, 11.6213) ccw
  line L319 (98.8485, 14.5379) -> (93.8485, 19.5379) construction
  line L320 (92.7879, 18.4772) -> (97.7879, 13.4772)
  arc A181 (97.7879, 13.4772) -> (99.9092, 15.5985) centre (98.8485, 14.5379) ccw
  line L321 (99.9092, 15.5985) -> (94.9092, 20.5985)
  arc A182 (94.9092, 20.5985) -> (92.7879, 18.4772) centre (93.8485, 19.5379) ccw
  line L322 (90.7879, 22.5985) -> (92.7879, 20.5985) construction
  line L323 (93.2879, 25.0985) -> (88.2879, 20.0985)
  arc A183 (86.1665, 22.2198) -> (88.2879, 20.0985) centre (87.2272, 21.1592) ccw
  line L324 (92.2272, 26.1592) -> (87.2272, 21.1592) construction
  line L325 (86.1665, 22.2198) -> (91.1665, 27.2198)
  arc A184 (93.2879, 25.0985) -> (91.1665, 27.2198) centre (92.2272, 26.1592) ccw
  line L326 (98.8485, 29.0757) -> (93.8485, 34.0757) construction
  line L327 (92.7879, 33.0151) -> (97.7879, 28.0151)
  arc A185 (97.7879, 28.0151) -> (99.9092, 30.1364) centre (98.8485, 29.0757) ccw
  line L328 (99.9092, 30.1364) -> (94.9092, 35.1364)
  arc A186 (94.9092, 35.1364) -> (92.7879, 33.0151) centre (93.8485, 34.0757) ccw
  line L329 (90.7879, 37.1364) -> (92.7879, 35.1364) construction
  line L330 (93.2879, 39.6364) -> (88.2879, 34.6364)
  arc A187 (86.1665, 36.7577) -> (88.2879, 34.6364) centre (87.2272, 35.6971) ccw
  line L331 (92.2272, 40.6971) -> (87.2272, 35.6971) construction
  line L332 (86.1665, 36.7577) -> (91.1665, 41.7577)
  arc A188 (93.2879, 39.6364) -> (91.1665, 41.7577) centre (92.2272, 40.6971) ccw
  line L333 (98.8485, 43.6136) -> (93.8485, 48.6136) construction
  line L334 (92.7879, 47.5529) -> (97.7879, 42.5529)
  arc A189 (97.7879, 42.5529) -> (99.9092, 44.6743) centre (98.8485, 43.6136) ccw
  line L335 (99.9092, 44.6743) -> (94.9092, 49.6743)
  arc A190 (94.9092, 49.6743) -> (92.7879, 47.5529) centre (93.8485, 48.6136) ccw
  line L336 (90.7879, 51.6743) -> (92.7879, 49.6743) construction
  line L337 (93.2879, 54.1743) -> (88.2879, 49.1743)
  arc A191 (86.1665, 51.2956) -> (88.2879, 49.1743) centre (87.2272, 50.2349) ccw
  line L338 (92.2272, 55.2349) -> (87.2272, 50.2349) construction
  line L339 (86.1665, 51.2956) -> (91.1665, 56.2956)
  arc A192 (93.2879, 54.1743) -> (91.1665, 56.2956) centre (92.2272, 55.2349) ccw
  line L340 (98.8485, 58.1515) -> (93.8485, 63.1515) construction
  line L341 (92.7879, 62.0908) -> (97.7879, 57.0908)
  arc A193 (97.7879, 57.0908) -> (99.9092, 59.2121) centre (98.8485, 58.1515) ccw
  line L342 (99.9092, 59.2121) -> (94.9092, 64.2121)
  arc A194 (94.9092, 64.2121) -> (92.7879, 62.0908) centre (93.8485, 63.1515) ccw
  line L343 (90.7879, 66.2121) -> (92.7879, 64.2121) construction
  line L344 (93.2879, 68.7121) -> (88.2879, 63.7121)
  arc A195 (86.1665, 65.8335) -> (88.2879, 63.7121) centre (87.2272, 64.7728) ccw
  line L345 (92.2272, 69.7728) -> (87.2272, 64.7728) construction
  line L346 (86.1665, 65.8335) -> (91.1665, 70.8335)
  arc A196 (93.2879, 68.7121) -> (91.1665, 70.8335) centre (92.2272, 69.7728) ccw
  line L347 (98.8485, 72.6893) -> (93.8485, 77.6893) construction
  line L348 (92.7879, 76.6287) -> (97.7879, 71.6287)
  arc A197 (97.7879, 71.6287) -> (99.9092, 73.75) centre (98.8485, 72.6893) ccw
  line L349 (99.9092, 73.75) -> (94.9092, 78.75)
  arc A198 (94.9092, 78.75) -> (92.7879, 76.6287) centre (93.8485, 77.6893) ccw
  line L350 (90.7879, 80.75) -> (92.7879, 78.75) construction
  line L351 (93.2879, 83.25) -> (88.2879, 78.25)
  arc A199 (86.1665, 80.3713) -> (88.2879, 78.25) centre (87.2272, 79.3107) ccw
  line L352 (92.2272, 84.3107) -> (87.2272, 79.3107) construction
  line L353 (86.1665, 80.3713) -> (91.1665, 85.3713)
  arc A200 (93.2879, 83.25) -> (91.1665, 85.3713) centre (92.2272, 84.3107) ccw
  line L354 (98.8485, 87.2272) -> (93.8485, 92.2272) construction
  line L355 (92.7879, 91.1665) -> (97.7879, 86.1665)
  arc A201 (97.7879, 86.1665) -> (99.9092, 88.2879) centre (98.8485, 87.2272) ccw
  line L356 (99.9092, 88.2879) -> (94.9092, 93.2879)
  arc A202 (94.9092, 93.2879) -> (92.7879, 91.1665) centre (93.8485, 92.2272) ccw
  line L357 (90.7879, 95.2879) -> (92.7879, 93.2879) construction
  line L358 (93.2879, 97.7879) -> (88.2879, 92.7879)
  arc A203 (86.1665, 94.9092) -> (88.2879, 92.7879) centre (87.2272, 93.8485) ccw
  line L359 (92.2272, 98.8485) -> (87.2272, 93.8485) construction
  line L360 (86.1665, 94.9092) -> (91.1665, 99.9092)
  arc A204 (93.2879, 97.7879) -> (91.1665, 99.9092) centre (92.2272, 98.8485) ccw
  line L361 (98.8485, 101.7651) -> (93.8485, 106.7651) construction
  line L362 (92.7879, 105.7044) -> (97.7879, 100.7044)
  arc A205 (97.7879, 100.7044) -> (99.9092, 102.8257) centre (98.8485, 101.7651) ccw
  line L363 (99.9092, 102.8257) -> (94.9092, 107.8257)
  arc A206 (94.9092, 107.8257) -> (92.7879, 105.7044) centre (93.8485, 106.7651) ccw
  line L364 (90.7879, 109.8257) -> (92.7879, 107.8257) construction
  line L365 (93.2879, 112.3257) -> (88.2879, 107.3257)
  arc A207 (86.1665, 109.4471) -> (88.2879, 107.3257) centre (87.2272, 108.3864) ccw
  line L366 (92.2272, 113.3864) -> (87.2272, 108.3864) construction
  line L367 (86.1665, 109.4471) -> (91.1665, 114.4471)
  arc A208 (93.2879, 112.3257) -> (91.1665, 114.4471) centre (92.2272, 113.3864) ccw
  line L368 (98.8485, 116.3029) -> (93.8485, 121.3029) construction
  line L369 (92.7879, 120.2423) -> (97.7879, 115.2423)
  arc A209 (97.7879, 115.2423) -> (99.9092, 117.3636) centre (98.8485, 116.3029) ccw
  line L370 (99.9092, 117.3636) -> (94.9092, 122.3636)
  arc A210 (94.9092, 122.3636) -> (92.7879, 120.2423) centre (93.8485, 121.3029) ccw
  line L371 (90.7879, 124.3636) -> (92.7879, 122.3636) construction
  line L372 (93.2879, 126.8636) -> (88.2879, 121.8636)
  arc A211 (86.1665, 123.9849) -> (88.2879, 121.8636) centre (87.2272, 122.9243) ccw
  line L373 (92.2272, 127.9243) -> (87.2272, 122.9243) construction
  line L374 (86.1665, 123.9849) -> (91.1665, 128.9849)
  arc A212 (93.2879, 126.8636) -> (91.1665, 128.9849) centre (92.2272, 127.9243) ccw
  line L375 (98.8485, 130.8408) -> (93.8485, 135.8408) construction
  line L376 (92.7879, 134.7802) -> (97.7879, 129.7802)
  arc A213 (97.7879, 129.7802) -> (99.9092, 131.9015) centre (98.8485, 130.8408) ccw
  line L377 (99.9092, 131.9015) -> (94.9092, 136.9015)
  arc A214 (94.9092, 136.9015) -> (92.7879, 134.7802) centre (93.8485, 135.8408) ccw
  line L378 (90.7879, 138.9015) -> (92.7879, 136.9015) construction
  line L379 (93.2879, 141.4015) -> (88.2879, 136.4015)
  arc A215 (86.1665, 138.5228) -> (88.2879, 136.4015) centre (87.2272, 137.4621) ccw
  line L380 (92.2272, 142.4621) -> (87.2272, 137.4621) construction
  line L381 (86.1665, 138.5228) -> (91.1665, 143.5228)
  arc A216 (93.2879, 141.4015) -> (91.1665, 143.5228) centre (92.2272, 142.4621) ccw
  line L382 (98.8485, 145.3787) -> (93.8485, 150.3787) construction
  line L383 (92.7879, 149.318) -> (97.7879, 144.318)
  arc A217 (97.7879, 144.318) -> (99.9092, 146.4393) centre (98.8485, 145.3787) ccw
  line L384 (99.9092, 146.4393) -> (94.9092, 151.4393)
  arc A218 (94.9092, 151.4393) -> (92.7879, 149.318) centre (93.8485, 150.3787) ccw
  line L385 (90.7879, 153.4393) -> (92.7879, 151.4393) construction
  line L386 (93.2879, 155.9393) -> (88.2879, 150.9393)
  arc A219 (86.1665, 153.0607) -> (88.2879, 150.9393) centre (87.2272, 152) ccw
  line L387 (92.2272, 157) -> (87.2272, 152) construction
  line L388 (86.1665, 153.0607) -> (91.1665, 158.0607)
  arc A220 (93.2879, 155.9393) -> (91.1665, 158.0607) centre (92.2272, 157) ccw
  line L389 (84.3107, 0) -> (79.3107, 5) construction
  line L390 (78.25, 3.9393) -> (83.25, -1.0607)
  arc A221 (83.25, -1.0607) -> (85.3713, 1.0607) centre (84.3107, 0) ccw
  line L391 (85.3713, 1.0607) -> (80.3713, 6.0607)
  arc A222 (80.3713, 6.0607) -> (78.25, 3.9393) centre (79.3107, 5) ccw
  line L392 (76.25, 8.0607) -> (78.25, 6.0607) construction
  line L393 (78.75, 10.5607) -> (73.75, 5.5607)
  arc A223 (71.6287, 7.682) -> (73.75, 5.5607) centre (72.6893, 6.6213) ccw
  line L394 (77.6893, 11.6213) -> (72.6893, 6.6213) construction
  line L395 (71.6287, 7.682) -> (76.6287, 12.682)
  arc A224 (78.75, 10.5607) -> (76.6287, 12.682) centre (77.6893, 11.6213) ccw
  line L396 (84.3107, 14.5379) -> (79.3107, 19.5379) construction
  line L397 (78.25, 18.4772) -> (83.25, 13.4772)
  arc A225 (83.25, 13.4772) -> (85.3713, 15.5985) centre (84.3107, 14.5379) ccw
  line L398 (85.3713, 15.5985) -> (80.3713, 20.5985)
  arc A226 (80.3713, 20.5985) -> (78.25, 18.4772) centre (79.3107, 19.5379) ccw
  line L399 (76.25, 22.5985) -> (78.25, 20.5985) construction
  line L400 (78.75, 25.0985) -> (73.75, 20.0985)
  arc A227 (71.6287, 22.2198) -> (73.75, 20.0985) centre (72.6893, 21.1592) ccw
  line L401 (77.6893, 26.1592) -> (72.6893, 21.1592) construction
  line L402 (71.6287, 22.2198) -> (76.6287, 27.2198)
  arc A228 (78.75, 25.0985) -> (76.6287, 27.2198) centre (77.6893, 26.1592) ccw
  line L403 (84.3107, 29.0757) -> (79.3107, 34.0757) construction
  line L404 (78.25, 33.0151) -> (83.25, 28.0151)
  arc A229 (83.25, 28.0151) -> (85.3713, 30.1364) centre (84.3107, 29.0757) ccw
  line L405 (85.3713, 30.1364) -> (80.3713, 35.1364)
  arc A230 (80.3713, 35.1364) -> (78.25, 33.0151) centre (79.3107, 34.0757) ccw
  line L406 (76.25, 37.1364) -> (78.25, 35.1364) construction
  line L407 (78.75, 39.6364) -> (73.75, 34.6364)
  arc A231 (71.6287, 36.7577) -> (73.75, 34.6364) centre (72.6893, 35.6971) ccw
  line L408 (77.6893, 40.6971) -> (72.6893, 35.6971) construction
  line L409 (71.6287, 36.7577) -> (76.6287, 41.7577)
  arc A232 (78.75, 39.6364) -> (76.6287, 41.7577) centre (77.6893, 40.6971) ccw
  line L410 (84.3107, 43.6136) -> (79.3107, 48.6136) construction
  line L411 (78.25, 47.5529) -> (83.25, 42.5529)
  arc A233 (83.25, 42.5529) -> (85.3713, 44.6743) centre (84.3107, 43.6136) ccw
  line L412 (85.3713, 44.6743) -> (80.3713, 49.6743)
  arc A234 (80.3713, 49.6743) -> (78.25, 47.5529) centre (79.3107, 48.6136) ccw
  line L413 (76.25, 51.6743) -> (78.25, 49.6743) construction
  line L414 (78.75, 54.1743) -> (73.75, 49.1743)
  arc A235 (71.6287, 51.2956) -> (73.75, 49.1743) centre (72.6893, 50.2349) ccw
  line L415 (77.6893, 55.2349) -> (72.6893, 50.2349) construction
  line L416 (71.6287, 51.2956) -> (76.6287, 56.2956)
  arc A236 (78.75, 54.1743) -> (76.6287, 56.2956) centre (77.6893, 55.2349) ccw
  line L417 (84.3107, 58.1515) -> (79.3107, 63.1515) construction
  line L418 (78.25, 62.0908) -> (83.25, 57.0908)
  arc A237 (83.25, 57.0908) -> (85.3713, 59.2121) centre (84.3107, 58.1515) ccw
  line L419 (85.3713, 59.2121) -> (80.3713, 64.2121)
  arc A238 (80.3713, 64.2121) -> (78.25, 62.0908) centre (79.3107, 63.1515) ccw
  line L420 (76.25, 66.2121) -> (78.25, 64.2121) construction
  line L421 (78.75, 68.7121) -> (73.75, 63.7121)
  arc A239 (71.6287, 65.8335) -> (73.75, 63.7121) centre (72.6893, 64.7728) ccw
  line L422 (77.6893, 69.7728) -> (72.6893, 64.7728) construction
  line L423 (71.6287, 65.8335) -> (76.6287, 70.8335)
  arc A240 (78.75, 68.7121) -> (76.6287, 70.8335) centre (77.6893, 69.7728) ccw
  line L424 (84.3107, 72.6893) -> (79.3107, 77.6893) construction
  line L425 (78.25, 76.6287) -> (83.25, 71.6287)
  arc A241 (83.25, 71.6287) -> (85.3713, 73.75) centre (84.3107, 72.6893) ccw
  line L426 (85.3713, 73.75) -> (80.3713, 78.75)
  arc A242 (80.3713, 78.75) -> (78.25, 76.6287) centre (79.3107, 77.6893) ccw
  line L427 (76.25, 80.75) -> (78.25, 78.75) construction
  line L428 (78.75, 83.25) -> (73.75, 78.25)
  arc A243 (71.6287, 80.3713) -> (73.75, 78.25) centre (72.6893, 79.3107) ccw
  line L429 (77.6893, 84.3107) -> (72.6893, 79.3107) construction
  line L430 (71.6287, 80.3713) -> (76.6287, 85.3713)
  arc A244 (78.75, 83.25) -> (76.6287, 85.3713) centre (77.6893, 84.3107) ccw
  line L431 (84.3107, 87.2272) -> (79.3107, 92.2272) construction
  line L432 (78.25, 91.1665) -> (83.25, 86.1665)
  arc A245 (83.25, 86.1665) -> (85.3713, 88.2879) centre (84.3107, 87.2272) ccw
  line L433 (85.3713, 88.2879) -> (80.3713, 93.2879)
  arc A246 (80.3713, 93.2879) -> (78.25, 91.1665) centre (79.3107, 92.2272) ccw
  line L434 (76.25, 95.2879) -> (78.25, 93.2879) construction
  line L435 (78.75, 97.7879) -> (73.75, 92.7879)
  arc A247 (71.6287, 94.9092) -> (73.75, 92.7879) centre (72.6893, 93.8485) ccw
  line L436 (77.6893, 98.8485) -> (72.6893, 93.8485) construction
  line L437 (71.6287, 94.9092) -> (76.6287, 99.9092)
  arc A248 (78.75, 97.7879) -> (76.6287, 99.9092) centre (77.6893, 98.8485) ccw
  line L438 (84.3107, 101.7651) -> (79.3107, 106.7651) construction
  line L439 (78.25, 105.7044) -> (83.25, 100.7044)
  arc A249 (83.25, 100.7044) -> (85.3713, 102.8257) centre (84.3107, 101.7651) ccw
  line L440 (85.3713, 102.8257) -> (80.3713, 107.8257)
  arc A250 (80.3713, 107.8257) -> (78.25, 105.7044) centre (79.3107, 106.7651) ccw
  line L441 (76.25, 109.8257) -> (78.25, 107.8257) construction
  line L442 (78.75, 112.3257) -> (73.75, 107.3257)
  arc A251 (71.6287, 109.4471) -> (73.75, 107.3257) centre (72.6893, 108.3864) ccw
  line L443 (77.6893, 113.3864) -> (72.6893, 108.3864) construction
  line L444 (71.6287, 109.4471) -> (76.6287, 114.4471)
  arc A252 (78.75, 112.3257) -> (76.6287, 114.4471) centre (77.6893, 113.3864) ccw
  line L445 (84.3107, 116.3029) -> (79.3107, 121.3029) construction
  line L446 (78.25, 120.2423) -> (83.25, 115.2423)
  arc A253 (83.25, 115.2423) -> (85.3713, 117.3636) centre (84.3107, 116.3029) ccw
  line L447 (85.3713, 117.3636) -> (80.3713, 122.3636)
  arc A254 (80.3713, 122.3636) -> (78.25, 120.2423) centre (79.3107, 121.3029) ccw
  line L448 (76.25, 124.3636) -> (78.25, 122.3636) construction
  line L449 (78.75, 126.8636) -> (73.75, 121.8636)
  arc A255 (71.6287, 123.9849) -> (73.75, 121.8636) centre (72.6893, 122.9243) ccw
  line L450 (77.6893, 127.9243) -> (72.6893, 122.9243) construction
  line L451 (71.6287, 123.9849) -> (76.6287, 128.9849)
  arc A256 (78.75, 126.8636) -> (76.6287, 128.9849) centre (77.6893, 127.9243) ccw
  line L452 (84.3107, 130.8408) -> (79.3107, 135.8408) construction
  line L453 (78.25, 134.7802) -> (83.25, 129.7802)
  arc A257 (83.25, 129.7802) -> (85.3713, 131.9015) centre (84.3107, 130.8408) ccw
  line L454 (85.3713, 131.9015) -> (80.3713, 136.9015)
  arc A258 (80.3713, 136.9015) -> (78.25, 134.7802) centre (79.3107, 135.8408) ccw